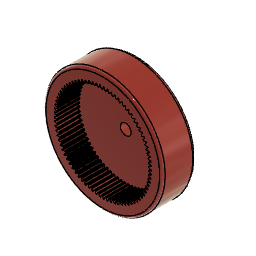
Aquazepp_Zahnkranz2 v37 (Autodesk Fusion 360 design; units mm, degrees)
description: Internal Gear; Module: 1.270000; Number of Teeth: 81; Pressure Angle: 20.000000; Root Fillet Radius: 0.040000; Clearance: 0.000000; Gear Thickness: 2.500000; Outer Diameter: 12.000000;
Autodesk Fusion 360 part; units mm, degrees
(part 1 of 3)
sketch "Skizze1" plane through (0, 0, 0) normal (0, 1, 0) x (1, 0, 0) in component "Internal Gear (81 teeth)"
  spline S0 degree 3 poles (38.2228, -33.6046) (38.0725, -33.5406) (37.9301, -33.4773) (37.7958, -33.4151) knots 0 0 0 0 1 1 1 1
  spline S1 degree 3 poles (40.3792, -34.3646) (39.532, -34.1197) (38.8155, -33.857) (38.2228, -33.6046) knots 0 0 0 0 1 1 1 1
  arc A0 (36.9675, -33.9106) -> (37.3302, -33.511) centre (0, 0) ccw
  arc A1 (36.9675, -33.9106) -> (36.9172, -34.3833) centre (37.2623, -34.181) ccw
  arc A2 (37.7958, -33.4151) -> (37.3302, -33.511) centre (37.6279, -33.7782) ccw
  spline S2 degree 3 poles (37.1472, -34.79) (37.4558, -35.3555) (37.7866, -36.0432) (38.1123, -36.8626) knots 0 0 0 0 1 1 1 1
  spline S3 degree 3 poles (37.5947, -37.3903) (36.7691, -37.0806) (36.0751, -36.7631) (35.5038, -36.4656) knots 0 0 0 0 1 1 1 1
  spline S4 degree 3 poles (36.9172, -34.3833) (36.9921, -34.511) (37.0689, -34.6465) (37.1472, -34.79) knots 0 0 0 0 1 1 1 1
  arc A3 (37.5947, -37.3903) -> (38.1123, -36.8626) centre (0, 0) ccw
  arc A4 (34.2285, -36.6734) -> (34.6211, -36.303) centre (0, 0) ccw
  arc A5 (31.2837, -39.2155) -> (31.161, -39.6748) centre (31.5331, -39.5282) ccw
  arc A6 (31.3657, -42.7504) -> (31.9586, -42.309) centre (0, 0) ccw
  spline S5 degree 3 poles (34.3395, -37.564) (34.6033, -38.1517) (34.8799, -38.863) (35.1411, -39.7052) knots 0 0 0 0 1 1 1 1
  arc A7 (28.1507, -41.5219) -> (27.9928, -41.9702) centre (28.3752, -41.8529) ccw
  spline S6 degree 3 poles (35.5038, -36.4656) (35.3588, -36.3901) (35.2218, -36.3159) (35.0927, -36.2435) knots 0 0 0 0 1 1 1 1
  arc A8 (34.5842, -40.1912) -> (35.1411, -39.7052) centre (0, 0) ccw
  arc A9 (28.1507, -41.5219) -> (28.5958, -41.2166) centre (0, 0) ccw
  spline S7 degree 3 poles (29.4428, -41.5136) (29.3112, -41.4166) (29.1873, -41.3222) (29.071, -41.2307) knots 0 0 0 0 1 1 1 1
  arc A10 (31.2837, -39.2155) -> (31.7038, -38.8767) centre (0, 0) ccw
  arc A11 (32.1786, -38.854) -> (31.7038, -38.8767) centre (31.9566, -39.1867) ccw
  spline S8 degree 3 poles (31.161, -39.6748) (31.2152, -39.8125) (31.2701, -39.9583) (31.3253, -40.1121) knots 0 0 0 0 1 1 1 1
  spline S9 degree 3 poles (34.1418, -37.1407) (34.2065, -37.2738) (34.2726, -37.4149) (34.3395, -37.564) knots 0 0 0 0 1 1 1 1
  arc A12 (35.0927, -36.2435) -> (34.6211, -36.303) centre (34.8972, -36.5925) ccw
  spline S10 degree 3 poles (32.5712, -39.1072) (32.4326, -39.0207) (32.3017, -38.9361) (32.1786, -38.854) knots 0 0 0 0 1 1 1 1
  spline S11 degree 3 poles (31.3657, -42.7504) (30.5979, -42.3168) (29.9613, -41.8959) (29.4428, -41.5136) knots 0 0 0 0 1 1 1 1
  arc A13 (34.2285, -36.6734) -> (34.1418, -37.1407) centre (34.5015, -36.9658) ccw
  spline S12 degree 3 poles (27.9928, -41.9702) (28.0362, -42.1117) (28.0796, -42.2613) (28.1227, -42.419) knots 0 0 0 0 1 1 1 1
  spline S13 degree 3 poles (34.5842, -40.1912) (33.7851, -39.8184) (33.1178, -39.4481) (32.5712, -39.1072) knots 0 0 0 0 1 1 1 1
  spline S14 degree 3 poles (31.3253, -40.1121) (31.5428, -40.7185) (31.7634, -41.449) (31.9586, -42.309) knots 0 0 0 0 1 1 1 1
  arc A14 (29.071, -41.2307) -> (28.5958, -41.2166) centre (28.8238, -41.5452) ccw
  spline S15 degree 3 poles (26.1373, -43.6704) (26.0136, -43.5635) (25.8974, -43.4597) (25.7885, -43.3595) knots 0 0 0 0 1 1 1 1
  arc A15 (24.8484, -43.5785) -> (24.6562, -44.0132) centre (25.0466, -43.9259) ccw
  arc A16 (24.3833, -47.0835) -> (25.0372, -46.739) centre (0, 0) ccw
  arc A17 (25.7885, -43.3595) -> (25.3158, -43.3086) centre (25.5177, -43.6539) ccw
  spline S16 degree 3 poles (24.6562, -44.0132) (24.6885, -44.1577) (24.7203, -44.3102) (24.751, -44.4707) knots 0 0 0 0 1 1 1 1
  arc A18 (21.3967, -45.373) -> (21.1714, -45.7916) centre (21.5673, -45.7348) ccw
  arc A19 (27.9586, -45.0524) -> (28.5839, -44.6583) centre (0, 0) ccw
  spline S17 degree 3 poles (21.1714, -45.7916) (21.1924, -45.9381) (21.2122, -46.0926) (21.2304, -46.255) knots 0 0 0 0 1 1 1 1
  spline S18 degree 3 poles (24.751, -44.4707) (24.8722, -45.1034) (24.9773, -45.8593) (25.0372, -46.739) knots 0 0 0 0 1 1 1 1
  spline S19 degree 3 poles (27.9586, -45.0524) (27.2266, -44.5606) (26.6246, -44.0917) (26.1373, -43.6704) knots 0 0 0 0 1 1 1 1
  spline S20 degree 3 poles (28.1227, -42.419) (28.2926, -43.0404) (28.4559, -43.7858) (28.5839, -44.6583) knots 0 0 0 0 1 1 1 1
  arc A20 (24.8484, -43.5785) -> (25.3158, -43.3086) centre (0, 0) ccw
  spline S21 degree 3 poles (17.5592, -47.2945) (17.5688, -47.4422) (17.5766, -47.5978) (17.5822, -47.7611) knots 0 0 0 0 1 1 1 1
  spline S22 degree 3 poles (20.6613, -48.8314) (20.0142, -48.2325) (19.4918, -47.6761) (19.0754, -47.1846) knots 0 0 0 0 1 1 1 1
  spline S23 degree 3 poles (22.6745, -45.5645) (22.5595, -45.4483) (22.4517, -45.3359) (22.3509, -45.2276) knots 0 0 0 0 1 1 1 1
  spline S24 degree 3 poles (24.3833, -47.0835) (23.6917, -46.5365) (23.1277, -46.0223) (22.6745, -45.5645) knots 0 0 0 0 1 1 1 1
  arc A21 (21.3967, -45.373) -> (21.8836, -45.1402) centre (0, 0) ccw
  arc A22 (20.6613, -48.8314) -> (21.34, -48.5387) centre (0, 0) ccw
  spline S25 degree 3 poles (21.2304, -46.255) (21.3023, -46.8952) (21.3484, -47.6569) (21.34, -48.5387) knots 0 0 0 0 1 1 1 1
  arc A23 (22.3509, -45.2276) -> (21.8836, -45.1402) centre (22.0581, -45.5001) ccw
  arc A24 (17.8163, -46.8946) -> (17.5592, -47.2945) centre (17.9584, -47.2686) ccw
  arc A25 (17.8163, -46.8946) -> (18.3198, -46.7002) centre (0, 0) ccw
  arc A26 (8.8431, -52.28) -> (9.571, -52.1517) centre (0, 0) ccw
  arc A27 (10.3562, -49.0844) -> (10.0404, -49.4397) centre (10.4388, -49.4758) ccw
  arc A28 (6.5214, -49.7393) -> (6.1791, -50.0691) centre (6.5734, -50.1359) ccw
  spline S26 degree 3 poles (17.5822, -47.7611) (17.6042, -48.4049) (17.5912, -49.1679) (17.5145, -50.0464) knots 0 0 0 0 1 1 1 1
  spline S27 degree 3 poles (13.8415, -48.513) (13.8396, -48.661) (13.8353, -48.8167) (13.8282, -48.98) knots 0 0 0 0 1 1 1 1
  arc A29 (14.1288, -48.1342) -> (13.8415, -48.513) centre (14.2414, -48.5181) ccw
  arc A30 (11.3182, -49.1629) -> (10.8837, -48.9701) centre (10.9705, -49.3606) ccw
  spline S28 degree 3 poles (15.3616, -48.5209) (15.266, -48.3884) (15.1768, -48.2606) (15.0939, -48.138) knots 0 0 0 0 1 1 1 1
  spline S29 degree 3 poles (16.8151, -50.2857) (16.2164, -49.6384) (15.7387, -49.0432) (15.3616, -48.5209) knots 0 0 0 0 1 1 1 1
  arc A31 (10.3562, -49.0844) -> (10.8837, -48.9701) centre (0, 0) ccw
  spline S30 degree 3 poles (8.8431, -52.28) (8.3515, -51.5479) (7.9715, -50.8861) (7.6798, -50.3118) knots 0 0 0 0 1 1 1 1
  spline S31 degree 3 poles (12.8678, -51.4375) (12.321, -50.7457) (11.8909, -50.1154) (11.5554, -49.5654) knots 0 0 0 0 1 1 1 1
  spline S32 degree 3 poles (19.0754, -47.1846) (18.9698, -47.0599) (18.871, -46.9394) (18.7789, -46.8236) knots 0 0 0 0 1 1 1 1
  arc A32 (16.8151, -50.2857) -> (17.5145, -50.0464) centre (0, 0) ccw
  arc A33 (15.0939, -48.138) -> (14.6458, -47.9795) centre (14.7626, -48.362) ccw
  spline S33 degree 3 poles (13.8282, -48.98) (13.8002, -49.6236) (13.7282, -50.3833) (13.5836, -51.2532) knots 0 0 0 0 1 1 1 1
  arc A34 (14.1288, -48.1342) -> (14.6458, -47.9795) centre (0, 0) ccw
  spline S34 degree 3 poles (11.5554, -49.5654) (11.4703, -49.4259) (11.3914, -49.2916) (11.3182, -49.1629) knots 0 0 0 0 1 1 1 1
  spline S35 degree 3 poles (10.0404, -49.4397) (10.0271, -49.5871) (10.0108, -49.742) (9.991, -49.9043) knots 0 0 0 0 1 1 1 1
  arc A35 (12.8678, -51.4375) -> (13.5836, -51.2532) centre (0, 0) ccw
  spline S36 degree 3 poles (9.991, -49.9043) (9.9133, -50.5437) (9.7826, -51.2956) (9.571, -52.1517) knots 0 0 0 0 1 1 1 1
  spline S37 degree 3 poles (7.6798, -50.3118) (7.6057, -50.1661) (7.5374, -50.0261) (7.4744, -49.8921) knots 0 0 0 0 1 1 1 1
  arc A36 (7.4744, -49.8921) -> (7.0562, -49.6663) centre (7.1124, -50.0623) ccw
  arc A37 (18.7789, -46.8236) -> (18.3198, -46.7002) centre (18.4659, -47.0726) ccw
  arc A38 (46.1935, -20.2794) -> (45.7794, -20.5129) centre (46.1444, -20.6764) ccw
  spline S38 degree 3 poles (-8.0485, -50.2541) (-8.0745, -50.0928) (-8.0968, -49.9386) (-8.1159, -49.7918) knots 0 0 0 0 1 1 1 1
  spline S39 degree 3 poles (-3.4519, -52.9102) (-3.7614, -52.0844) (-3.9785, -51.3529) (-4.13, -50.7267) knots 0 0 0 0 1 1 1 1
  arc A39 (45.556, -21.0042) -> (45.7794, -20.5129) centre (0, 0) ccw
  arc A40 (44.4831, -23.7981) -> (44.0521, -23.9987) centre (44.4034, -24.1901) ccw
  arc A41 (43.7914, -24.4713) -> (44.0521, -23.9987) centre (0, 0) ccw
  spline S40 degree 3 poles (44.9423, -23.884) (44.7812, -23.8564) (44.6281, -23.8276) (44.4831, -23.7981) knots 0 0 0 0 1 1 1 1
  spline S41 degree 3 poles (4.7652, -52.8081) (4.3318, -52.0401) (4.0043, -51.3508) (3.7579, -50.7556) knots 0 0 0 0 1 1 1 1
  spline S42 degree 3 poles (47.2158, -24.1262) (46.335, -24.0833) (45.5772, -23.9929) (44.9423, -23.884) knots 0 0 0 0 1 1 1 1
  spline S43 degree 3 poles (6.1791, -50.0691) (6.1543, -50.215) (6.1261, -50.3682) (6.0938, -50.5284) knots 0 0 0 0 1 1 1 1
  arc A42 (-5.125, -49.9025) -> (-5.5342, -50.1445) centre (-5.1659, -50.3004) ccw
  spline S44 degree 3 poles (48.8097, -14.4179) (49.3392, -14.7847) (49.9435, -15.2507) (50.6023, -15.8369) knots 0 0 0 0 1 1 1 1
  spline S45 degree 3 poles (44.169, -25.2855) (44.5997, -25.7646) (45.0802, -26.3574) (45.5861, -27.0797) knots 0 0 0 0 1 1 1 1
  spline S46 degree 3 poles (43.8514, -24.9428) (43.9537, -25.0498) (44.0597, -25.164) (44.169, -25.2855) knots 0 0 0 0 1 1 1 1
  arc A43 (2.6474, -50.0951) -> (2.2805, -50.3974) centre (2.6685, -50.4945) ccw
  arc A44 (4.7652, -52.8081) -> (5.5009, -52.7365) centre (0, 0) ccw
  spline S47 degree 3 poles (-0.1866, -50.8942) (-0.2372, -50.7388) (-0.2831, -50.59) (-0.3246, -50.4479) knots 0 0 0 0 1 1 1 1
  arc A45 (-4.233, -50.271) -> (-4.5879, -49.9548) centre (-4.6244, -50.3531) ccw
  spline S48 degree 3 poles (6.0938, -50.5284) (5.9667, -51.16) (5.7781, -51.8994) (5.5009, -52.7365) knots 0 0 0 0 1 1 1 1
  arc A46 (-3.4519, -52.9102) -> (-2.714, -52.9531) centre (0, 0) ccw
  arc A47 (0.6587, -53.0186) -> (1.3977, -53.0042) centre (0, 0) ccw
  arc A48 (-5.125, -49.9025) -> (-4.5879, -49.9548) centre (0, 0) ccw
  spline S49 degree 3 poles (-1.787, -50.8632) (-2.0101, -51.4675) (-2.3107, -52.1689) (-2.714, -52.9531) knots 0 0 0 0 1 1 1 1
  spline S50 degree 3 poles (-5.7231, -50.5718) (-5.9924, -51.157) (-6.3465, -51.833) (-6.8093, -52.5836) knots 0 0 0 0 1 1 1 1
  arc A49 (47.2158, -24.1262) -> (47.5475, -23.4657) centre (0, 0) ccw
  arc A50 (45.2042, -27.7125) -> (45.5861, -27.0797) centre (0, 0) ccw
  spline S51 degree 3 poles (48.0931, -16.6527) (47.9296, -16.6503) (47.7739, -16.6455) (47.6261, -16.6388) knots 0 0 0 0 1 1 1 1
  arc A51 (47.0467, -17.4108) -> (47.1789, -17.8674) centre (47.4218, -17.5496) ccw
  arc A52 (43.7914, -24.4713) -> (43.8514, -24.9428) centre (44.1406, -24.6664) ccw
  arc A53 (42.5051, -27.1736) -> (42.0599, -27.3403) centre (42.3953, -27.5583) ccw
  arc A54 (-0.3246, -50.4479) -> (-0.703, -50.1601) centre (-0.7086, -50.56) ccw
  spline S52 degree 3 poles (-4.13, -50.7267) (-4.1684, -50.5679) (-4.2026, -50.4159) (-4.233, -50.271) knots 0 0 0 0 1 1 1 1
  spline S53 degree 3 poles (-7.5416, -52.4836) (-7.7862, -51.6363) (-7.946, -50.8901) (-8.0485, -50.2541) knots 0 0 0 0 1 1 1 1
  arc A55 (-8.9767, -49.3553) -> (-8.4452, -49.449) centre (0, 0) ccw
  spline S54 degree 3 poles (50.3766, -16.5407) (49.4998, -16.6345) (48.7372, -16.6622) (48.0931, -16.6527) knots 0 0 0 0 1 1 1 1
  spline S55 degree 3 poles (-5.5342, -50.1445) (-5.5919, -50.2807) (-5.6548, -50.4233) (-5.7231, -50.5718) knots 0 0 0 0 1 1 1 1
  arc A56 (45.556, -21.0042) -> (45.6525, -21.4697) centre (45.9193, -21.1717) ccw
  arc A57 (6.5214, -49.7393) -> (7.0562, -49.6663) centre (0, 0) ccw
  arc A58 (-8.1159, -49.7918) -> (-8.4452, -49.449) centre (-8.5125, -49.8433) ccw
  spline S56 degree 3 poles (48.9434, -20.3948) (48.0619, -20.4203) (47.2994, -20.3889) (46.658, -20.3295) knots 0 0 0 0 1 1 1 1
  spline S57 degree 3 poles (45.9956, -21.7867) (46.4621, -22.231) (46.9871, -22.7848) (47.5475, -23.4657) knots 0 0 0 0 1 1 1 1
  spline S58 degree 3 poles (48.4216, -14.1576) (48.5458, -14.2382) (48.6753, -14.3248) (48.8097, -14.4179) knots 0 0 0 0 1 1 1 1
  spline S59 degree 3 poles (2.1599, -50.8487) (1.9843, -51.4685) (1.7389, -52.1911) (1.3977, -53.0042) knots 0 0 0 0 1 1 1 1
  arc A59 (50.3766, -16.5407) -> (50.6023, -15.8369) centre (0, 0) ccw
  spline S60 degree 3 poles (46.658, -20.3295) (46.4952, -20.3145) (46.3404, -20.2976) (46.1935, -20.2794) knots 0 0 0 0 1 1 1 1
  arc A60 (48.9434, -20.3948) -> (49.2229, -19.7105) centre (0, 0) ccw
  spline S61 degree 3 poles (-1.6318, -50.4225) (-1.6788, -50.5629) (-1.7304, -50.7099) (-1.787, -50.8632) knots 0 0 0 0 1 1 1 1
  arc A61 (-1.2426, -50.1496) -> (-0.703, -50.1601) centre (0, 0) ccw
  arc A62 (2.6474, -50.0951) -> (3.1862, -50.0637) centre (0, 0) ccw
  arc A63 (3.5857, -50.3213) -> (3.1862, -50.0637) centre (3.2116, -50.4629) ccw
  arc A64 (-7.5416, -52.4836) -> (-6.8093, -52.5836) centre (0, 0) ccw
  spline S62 degree 3 poles (0.6587, -53.0186) (0.2861, -52.2193) (0.0129, -51.5067) (-0.1866, -50.8942) knots 0 0 0 0 1 1 1 1
  arc A65 (-8.9767, -49.3553) -> (-9.4034, -49.5648) centre (-9.0483, -49.7489) ccw
  arc A66 (47.6261, -16.6388) -> (47.2313, -16.9036) centre (47.6079, -17.0384) ccw
  spline S63 degree 3 poles (2.2805, -50.3974) (2.2445, -50.5409) (2.2045, -50.6915) (2.1599, -50.8487) knots 0 0 0 0 1 1 1 1
  arc A67 (47.0467, -17.4108) -> (47.2313, -16.9036) centre (0, 0) ccw
  spline S64 degree 3 poles (45.6525, -21.4697) (45.7627, -21.5684) (45.8773, -21.674) (45.9956, -21.7867) knots 0 0 0 0 1 1 1 1
  arc A68 (-1.2426, -50.1496) -> (-1.6318, -50.4225) centre (-1.2525, -50.5495) ccw
  spline S65 degree 3 poles (3.7579, -50.7556) (3.6953, -50.6046) (3.6381, -50.4598) (3.5857, -50.3213) knots 0 0 0 0 1 1 1 1
  spline S66 degree 3 poles (47.1789, -17.8674) (47.2965, -17.9573) (47.4189, -18.0537) (47.5456, -18.1569) knots 0 0 0 0 1 1 1 1
  spline S67 degree 3 poles (47.5456, -18.1569) (48.0451, -18.5637) (48.6115, -19.0751) (49.2229, -19.7105) knots 0 0 0 0 1 1 1 1
  spline S68 degree 3 poles (-48.2139, 16.2996) (-48.7288, 16.6867) (-49.3146, 17.1759) (-49.9502, 17.7871) knots 0 0 0 0 1 1 1 1
  arc A69 (-46.3362, 19.2219) -> (-46.5403, 18.7223) centre (0, 0) ccw
  spline S69 degree 3 poles (-38.2227, 32.926) (-38.3024, 33.0507) (-38.3844, 33.1831) (-38.4682, 33.3234) knots 0 0 0 0 1 1 1 1
  arc A70 (-39.0163, 35.9045) -> (-39.513, 35.3571) centre (0, 0) ccw
  spline S70 degree 3 poles (-44.0956, 29.4445) (-43.2258, 29.2997) (-42.4836, 29.1219) (-41.8657, 28.94) knots 0 0 0 0 1 1 1 1
  spline S71 degree 3 poles (-39.0163, 35.9045) (-38.1793, 35.627) (-37.4735, 35.3366) (-36.8911, 35.0615) knots 0 0 0 0 1 1 1 1
  spline S72 degree 3 poles (40.712, -30.5416) (40.5571, -30.4894) (40.4103, -30.4373) (40.2716, -30.3858) knots 0 0 0 0 1 1 1 1
  arc A71 (-46.2447, 25.9389) -> (-46.6018, 25.2917) centre (0, 0) ccw
  arc A72 (-47.6864, 15.5734) -> (-47.8363, 16.0246) centre (-48.0667, 15.6976) ccw
  arc A73 (-43.5268, 25.5051) -> (-43.0884, 25.6888) centre (-43.432, 25.8936) ccw
  spline S73 degree 3 poles (-41.6813, 32.773) (-40.8253, 32.5612) (-40.0992, 32.3265) (-39.4971, 32.0973) knots 0 0 0 0 1 1 1 1
  arc A74 (42.9207, -31.1322) -> (43.3505, -30.5308) centre (0, 0) ccw
  spline S74 degree 3 poles (-47.8363, 16.0246) (-47.9572, 16.1098) (-48.0832, 16.2014) (-48.2139, 16.2996) knots 0 0 0 0 1 1 1 1
  arc A75 (-44.7073, 22.7548) -> (-44.9495, 22.2725) centre (0, 0) ccw
  arc A76 (-38.2546, 32.4517) -> (-38.2227, 32.926) centre (-38.5596, 32.7105) ccw
  arc A77 (-39.0631, 31.9244) -> (-38.6015, 32.0383) centre (-38.9093, 32.2937) ccw
  arc A78 (-44.7073, 22.7548) -> (-44.7856, 23.2237) centre (-45.0638, 22.9363) ccw
  arc A79 (40.2716, -30.3858) -> (39.8148, -30.5174) centre (40.1323, -30.7607) ccw
  spline S75 degree 3 poles (-46.2447, 25.9389) (-45.3663, 25.8619) (-44.6126, 25.7422) (-43.9824, 25.6087) knots 0 0 0 0 1 1 1 1
  spline S76 degree 3 poles (-36.8911, 35.0615) (-36.7433, 34.9917) (-36.6035, 34.9229) (-36.4717, 34.8555) knots 0 0 0 0 1 1 1 1
  spline S77 degree 3 poles (39.7314, -31.8068) (40.0829, -32.3466) (40.466, -33.0066) (40.8543, -33.7984) knots 0 0 0 0 1 1 1 1
  spline S78 degree 3 poles (-46.8058, 19.9868) (-47.2892, 20.4127) (-47.8353, 20.9457) (-48.4216, 21.6044) knots 0 0 0 0 1 1 1 1
  spline S79 degree 3 poles (41.7867, -28.266) (41.8804, -28.3806) (41.9772, -28.5026) (42.0767, -28.6322) knots 0 0 0 0 1 1 1 1
  spline S80 degree 3 poles (-40.6593, 29.865) (-40.7484, 29.9831) (-40.8405, 30.1088) (-40.9349, 30.2422) knots 0 0 0 0 1 1 1 1
  arc A80 (-47.6864, 15.5734) -> (-47.8512, 15.0595) centre (0, 0) ccw
  arc A81 (-40.6543, 29.3897) -> (-40.6593, 29.865) centre (-40.9785, 29.624) ccw
  arc A82 (39.4842, -30.944) -> (39.8148, -30.5174) centre (0, 0) ccw
  arc A83 (-49.6974, 18.4817) -> (-49.9502, 17.7871) centre (0, 0) ccw
  spline S81 degree 3 poles (-49.6974, 18.4817) (-48.8176, 18.5413) (-48.0545, 18.5395) (-47.4112, 18.505) knots 0 0 0 0 1 1 1 1
  arc A84 (-41.4195, 28.8014) -> (-40.9682, 28.9506) centre (-41.2948, 29.1814) ccw
  spline S82 degree 3 poles (42.0767, -28.6322) (42.469, -29.1432) (42.9021, -29.7715) (43.3505, -30.5308) knots 0 0 0 0 1 1 1 1
  spline S83 degree 3 poles (-48.7026, 14.7754) (-48.5392, 14.7793) (-48.3834, 14.7806) (-48.2354, 14.7796) knots 0 0 0 0 1 1 1 1
  spline S84 degree 3 poles (-45.1162, 23.5538) (-45.5652, 24.0158) (-46.0683, 24.5896) (-46.6018, 25.2917) knots 0 0 0 0 1 1 1 1
  spline S85 degree 3 poles (-47.4112, 18.505) (-47.248, 18.4963) (-47.0926, 18.4855) (-46.9451, 18.473) knots 0 0 0 0 1 1 1 1
  arc A85 (-46.3362, 19.2219) -> (-46.4506, 19.6833) centre (-46.7057, 19.3752) ccw
  arc A86 (40.3792, -34.3646) -> (40.8543, -33.7984) centre (0, 0) ccw
  arc A87 (-42.8096, 26.1509) -> (-42.8513, 26.6244) centre (-43.1509, 26.3594) ccw
  arc A88 (-44.0956, 29.4445) -> (-44.5018, 28.8269) centre (0, 0) ccw
  spline S86 degree 3 poles (-43.1553, 26.9792) (-43.5671, 27.4746) (-44.0243, 28.0856) (-44.5018, 28.8269) knots 0 0 0 0 1 1 1 1
  spline S87 degree 3 poles (-42.8513, 26.6244) (-42.9494, 26.7353) (-43.0509, 26.8535) (-43.1553, 26.9792) knots 0 0 0 0 1 1 1 1
  arc A89 (-45.3724, 22.0554) -> (-44.9495, 22.2725) centre (-45.308, 22.4501) ccw
  spline S88 degree 3 poles (-44.7856, 23.2237) (-44.892, 23.3266) (-45.0023, 23.4366) (-45.1162, 23.5538) knots 0 0 0 0 1 1 1 1
  spline S89 degree 3 poles (-41.8657, 28.94) (-41.7089, 28.8939) (-41.5601, 28.8475) (-41.4195, 28.8014) knots 0 0 0 0 1 1 1 1
  spline S90 degree 3 poles (42.9563, -27.2949) (42.7979, -27.2549) (42.6475, -27.2143) (42.5051, -27.1736) knots 0 0 0 0 1 1 1 1
  arc A90 (41.7634, -27.7912) -> (42.0599, -27.3403) centre (0, 0) ccw
  arc A91 (-40.6543, 29.3897) -> (-40.9682, 28.9506) centre (0, 0) ccw
  arc A92 (-42.8096, 26.1509) -> (-43.0884, 25.6888) centre (0, 0) ccw
  spline S91 degree 3 poles (-46.4506, 19.6833) (-46.5646, 19.7777) (-46.6832, 19.8788) (-46.8058, 19.9868) knots 0 0 0 0 1 1 1 1
  arc A93 (41.7634, -27.7912) -> (41.7867, -28.266) centre (42.0964, -28.0128) ccw
  spline S92 degree 3 poles (42.9207, -31.1322) (42.0572, -30.9537) (41.3225, -30.7473) (40.712, -30.5416) knots 0 0 0 0 1 1 1 1
  arc A94 (-48.1157, 22.2773) -> (-48.4216, 21.6044) centre (0, 0) ccw
  arc A95 (-48.2354, 14.7796) -> (-47.8512, 15.0595) centre (-48.2328, 15.1796) ccw
  spline S93 degree 3 poles (-45.8346, 22.1234) (-45.6726, 22.102) (-45.5185, 22.0792) (-45.3724, 22.0554) knots 0 0 0 0 1 1 1 1
  spline S94 degree 3 poles (-48.1157, 22.2773) (-47.234, 22.2686) (-46.4733, 22.2076) (-45.8346, 22.1234) knots 0 0 0 0 1 1 1 1
  spline S95 degree 3 poles (-43.9824, 25.6087) (-43.8225, 25.5749) (-43.6706, 25.5401) (-43.5268, 25.5051) knots 0 0 0 0 1 1 1 1
  spline S96 degree 3 poles (-40.9349, 30.2422) (-41.307, 30.7681) (-41.7155, 31.4127) (-42.1341, 32.1888) knots 0 0 0 0 1 1 1 1
  arc A96 (-46.9451, 18.473) -> (-46.5403, 18.7223) centre (-46.9114, 18.8716) ccw
  arc A97 (-41.6813, 32.773) -> (-42.1341, 32.1888) centre (0, 0) ccw
  spline S97 degree 3 poles (-39.4971, 32.0973) (-39.3444, 32.0391) (-39.1997, 31.9813) (-39.0631, 31.9244) knots 0 0 0 0 1 1 1 1
  arc A98 (-38.2546, 32.4517) -> (-38.6015, 32.0383) centre (0, 0) ccw
  arc A99 (39.4842, -30.944) -> (39.4706, -31.4191) centre (39.799, -31.1907) ccw
  spline S98 degree 3 poles (45.2042, -27.7125) (44.3294, -27.6015) (43.5809, -27.4527) (42.9563, -27.2949) knots 0 0 0 0 1 1 1 1
  spline S99 degree 3 poles (39.4706, -31.4191) (39.5552, -31.5406) (39.6423, -31.6698) (39.7314, -31.8068) knots 0 0 0 0 1 1 1 1
  spline S100 degree 3 poles (-13.4687, 49.0801) (-13.3782, 48.9439) (-13.2941, 48.8128) (-13.216, 48.6871) knots 0 0 0 0 1 1 1 1
  arc A100 (-12.2517, 48.6459) -> (-11.9499, 49.0132) centre (-12.3494, 49.0338) ccw
  spline S101 degree 3 poles (-14.8527, 50.8999) (-14.2794, 50.2298) (-13.8252, 49.6166) (-13.4687, 49.0801) knots 0 0 0 0 1 1 1 1
  arc A101 (-33.661, 37.577) -> (-33.1874, 37.6181) centre (-33.452, 37.9181) ccw
  spline S102 degree 3 poles (-29.7464, 41.2966) (-29.9402, 41.9109) (-30.1323, 42.6495) (-30.294, 43.5164) knots 0 0 0 0 1 1 1 1
  arc A102 (-14.8527, 50.8999) -> (-15.5607, 50.6879) centre (0, 0) ccw
  arc A103 (-13.216, 48.6871) -> (-12.7744, 48.5113) centre (-12.8762, 48.8981) ccw
  arc A104 (-35.6248, 35.3186) -> (-36.0027, 34.9332) centre (0, 0) ccw
  arc A105 (-26.5195, 42.5822) -> (-26.3443, 43.0241) centre (-26.731, 42.9217) ccw
  spline S103 degree 3 poles (-35.7702, 36.2042) (-36.0567, 36.7813) (-36.3606, 37.4812) (-36.6543, 38.3127) knots 0 0 0 0 1 1 1 1
  arc A106 (-29.7396, 40.3991) -> (-30.1725, 40.0768) centre (0, 0) ccw
  arc A107 (-18.7523, 49.5959) -> (-19.4419, 49.3297) centre (0, 0) ccw
  arc A108 (-12.2517, 48.6459) -> (-12.7744, 48.5113) centre (0, 0) ccw
  arc A109 (-10.8636, 51.8978) -> (-11.586, 51.7413) centre (0, 0) ccw
  spline S104 degree 3 poles (-11.9499, 49.0132) (-11.9423, 49.161) (-11.932, 49.3164) (-11.9186, 49.4793) knots 0 0 0 0 1 1 1 1
  arc A110 (-9.4034, 49.5648) -> (-8.9767, 49.3553) centre (-9.0483, 49.7489) ccw
  spline S105 degree 3 poles (-11.9186, 49.4793) (-11.8657, 50.1213) (-11.7642, 50.8777) (-11.586, 51.7413) knots 0 0 0 0 1 1 1 1
  spline S106 degree 3 poles (-29.5991, 40.8532) (-29.648, 40.9929) (-29.6972, 41.1407) (-29.7464, 41.2966) knots 0 0 0 0 1 1 1 1
  arc A111 (-29.7396, 40.3991) -> (-29.5991, 40.8532) centre (-29.9767, 40.7212) ccw
  spline S107 degree 3 poles (-32.9998, 41.502) (-32.2157, 41.0985) (-31.5633, 40.7026) (-31.0303, 40.3407) knots 0 0 0 0 1 1 1 1
  arc A112 (-32.7808, 37.973) -> (-33.1874, 37.6181) centre (0, 0) ccw
  spline S108 degree 3 poles (-26.3443, 43.0241) (-26.3822, 43.1672) (-26.4198, 43.3183) (-26.4568, 43.4775) knots 0 0 0 0 1 1 1 1
  spline S109 degree 3 poles (-27.8109, 42.624) (-27.6832, 42.522) (-27.5631, 42.4229) (-27.4504, 42.327) knots 0 0 0 0 1 1 1 1
  spline S110 degree 3 poles (-38.4682, 33.3234) (-38.7985, 33.8765) (-39.1558, 34.5509) (-39.513, 35.3571) knots 0 0 0 0 1 1 1 1
  arc A113 (-26.5195, 42.5822) -> (-26.9761, 42.2944) centre (0, 0) ccw
  spline S111 degree 3 poles (-26.4568, 43.4775) (-26.6024, 44.105) (-26.7367, 44.8563) (-26.8307, 45.7331) knots 0 0 0 0 1 1 1 1
  arc A114 (-36.4717, 34.8555) -> (-36.0027, 34.9332) centre (-36.2898, 35.2118) ccw
  arc A115 (-24.0878, 44.3269) -> (-23.6175, 44.2577) centre (-23.8058, 44.6106) ccw
  arc A116 (-23.14, 44.5092) -> (-22.931, 44.9362) centre (-23.3245, 44.8641) ccw
  spline S112 degree 3 poles (-22.5393, 47.9936) (-21.8694, 47.4201) (-21.3258, 46.8845) (-20.8907, 46.4094) knots 0 0 0 0 1 1 1 1
  arc A117 (-32.7808, 37.973) -> (-32.6759, 38.4367) centre (-33.0422, 38.2758) ccw
  arc A118 (-36.1166, 38.82) -> (-36.6543, 38.3127) centre (0, 0) ccw
  spline S113 degree 3 poles (-32.6759, 38.4367) (-32.7355, 38.5722) (-32.796, 38.7157) (-32.8571, 38.8673) knots 0 0 0 0 1 1 1 1
  spline S114 degree 3 poles (-32.8571, 38.8673) (-33.098, 39.4648) (-33.3467, 40.1862) (-33.5751, 41.0379) knots 0 0 0 0 1 1 1 1
  spline S115 degree 3 poles (-19.3799, 46.578) (-19.3952, 46.7253) (-19.409, 46.8804) (-19.4209, 47.0434) knots 0 0 0 0 1 1 1 1
  spline S116 degree 3 poles (-18.7523, 49.5959) (-18.1289, 48.9722) (-17.6285, 48.3961) (-17.2315, 47.8887) knots 0 0 0 0 1 1 1 1
  spline S117 degree 3 poles (-31.0303, 40.3407) (-30.8951, 40.2489) (-30.7677, 40.1594) (-30.6478, 40.0725) knots 0 0 0 0 1 1 1 1
  arc A119 (-29.6845, 43.9344) -> (-30.294, 43.5164) centre (0, 0) ccw
  spline S118 degree 3 poles (-34.0631, 37.8148) (-33.9212, 37.7338) (-33.7872, 37.6543) (-33.661, 37.577) knots 0 0 0 0 1 1 1 1
  spline S119 degree 3 poles (-29.6845, 43.9344) (-28.934, 43.4714) (-28.3142, 43.0261) (-27.8109, 42.624) knots 0 0 0 0 1 1 1 1
  arc A120 (-27.4504, 42.327) -> (-26.9761, 42.2944) centre (-27.1912, 42.6317) ccw
  arc A121 (-22.5393, 47.9936) -> (-23.2061, 47.6747) centre (0, 0) ccw
  spline S120 degree 3 poles (-19.4209, 47.0434) (-19.4679, 47.6859) (-19.4845, 48.4489) (-19.4419, 49.3297) knots 0 0 0 0 1 1 1 1
  arc A122 (-26.1906, 46.1026) -> (-26.8307, 45.7331) centre (0, 0) ccw
  arc A123 (-20.5804, 46.0602) -> (-20.1168, 45.9548) centre (-20.2772, 46.3212) ccw
  arc A124 (-23.14, 44.5092) -> (-23.6175, 44.2577) centre (0, 0) ccw
  arc A125 (-30.6478, 40.0725) -> (-30.1725, 40.0768) centre (-30.4131, 40.3963) ccw
  spline S121 degree 3 poles (-36.1166, 38.82) (-35.3037, 38.4784) (-34.6225, 38.1343) (-34.0631, 37.8148) knots 0 0 0 0 1 1 1 1
  arc A126 (-35.6248, 35.3186) -> (-35.5562, 35.7889) centre (-35.9089, 35.6002) ccw
  spline S122 degree 3 poles (-26.1906, 46.1026) (-25.4783, 45.5828) (-24.8949, 45.0909) (-24.4243, 44.651) knots 0 0 0 0 1 1 1 1
  arc A127 (-32.9998, 41.502) -> (-33.5751, 41.0379) centre (0, 0) ccw
  arc A128 (-19.6213, 46.1685) -> (-19.3799, 46.578) centre (-19.7777, 46.5367) ccw
  spline S123 degree 3 poles (-20.8907, 46.4094) (-20.7803, 46.2889) (-20.6769, 46.1724) (-20.5804, 46.0602) knots 0 0 0 0 1 1 1 1
  arc A129 (-19.6213, 46.1685) -> (-20.1168, 45.9548) centre (0, 0) ccw
  spline S124 degree 3 poles (-24.4243, 44.651) (-24.3048, 44.5394) (-24.1928, 44.4312) (-24.0878, 44.3269) knots 0 0 0 0 1 1 1 1
  spline S125 degree 3 poles (-35.5562, 35.7889) (-35.6261, 35.9194) (-35.6976, 36.0578) (-35.7702, 36.2042) knots 0 0 0 0 1 1 1 1
  spline S126 degree 3 poles (-22.931, 44.9362) (-22.9577, 45.0818) (-22.9835, 45.2354) (-23.008, 45.397) knots 0 0 0 0 1 1 1 1
  arc A130 (-15.9846, 47.5502) -> (-15.7122, 47.9398) centre (-16.112, 47.9294) ccw
  spline S127 degree 3 poles (-17.2315, 47.8887) (-17.1308, 47.76) (-17.0368, 47.6358) (-16.9492, 47.5165) knots 0 0 0 0 1 1 1 1
  arc A131 (-16.9492, 47.5165) -> (-16.4952, 47.3755) centre (-16.6267, 47.7532) ccw
  arc A132 (-15.9846, 47.5502) -> (-16.4952, 47.3755) centre (0, 0) ccw
  spline S128 degree 3 poles (-15.717, 48.4069) (-15.714, 49.0511) (-15.6715, 49.8131) (-15.5607, 50.6879) knots 0 0 0 0 1 1 1 1
  spline S129 degree 3 poles (-15.7122, 47.9398) (-15.716, 48.0877) (-15.7178, 48.2435) (-15.717, 48.4069) knots 0 0 0 0 1 1 1 1
  spline S130 degree 3 poles (-23.008, 45.397) (-23.1046, 46.0339) (-23.1803, 46.7933) (-23.2061, 47.6747) knots 0 0 0 0 1 1 1 1
  spline S131 degree 3 poles (-46.6018, -25.2917) (-46.0683, -24.5896) (-45.5652, -24.0158) (-45.1162, -23.5538) knots 0 0 0 0 1 1 1 1
  arc A133 (-49.9398, 7.1488) -> (-49.6035, 7.4847) centre (-49.999, 7.5444) ccw
  spline S132 degree 3 poles (-45.1162, -23.5538) (-45.0023, -23.4366) (-44.892, -23.3266) (-44.7856, -23.2237) knots 0 0 0 0 1 1 1 1
  arc A134 (-48.4216, -21.6044) -> (-48.1157, -22.2773) centre (0, 0) ccw
  spline S133 degree 3 poles (-48.4216, -21.6044) (-47.8353, -20.9457) (-47.2892, -20.4127) (-46.8058, -19.9868) knots 0 0 0 0 1 1 1 1
  spline S134 degree 3 poles (-45.8346, -22.1234) (-46.4733, -22.2076) (-47.234, -22.2686) (-48.1157, -22.2773) knots 0 0 0 0 1 1 1 1
  spline S135 degree 3 poles (-50.6732, 4.7414) (-51.2635, 4.9993) (-51.9463, 5.3402) (-52.7058, 5.7883) knots 0 0 0 0 1 1 1 1
  arc A135 (-46.4506, -19.6833) -> (-46.3362, -19.2219) centre (-46.7057, -19.3752) ccw
  arc A136 (-8.4452, 49.449) -> (-8.9767, 49.3553) centre (0, 0) ccw
  spline S136 degree 3 poles (-49.7011, 10.9569) (-49.5385, 10.9735) (-49.3833, 10.9868) (-49.2357, 10.9973) knots 0 0 0 0 1 1 1 1
  spline S137 degree 3 poles (-51.9563, 10.5805) (-51.0963, 10.7754) (-50.342, 10.8915) (-49.7011, 10.9569) knots 0 0 0 0 1 1 1 1
  arc A137 (-50.3437, 3.2573) -> (-50.0343, 3.6183) centre (-50.4333, 3.6472) ccw
  arc A138 (-48.7499, 11.8313) -> (-48.8743, 11.3061) centre (0, 0) ccw
  arc A139 (-46.5403, -18.7223) -> (-46.3362, -19.2219) centre (0, 0) ccw
  arc A140 (-46.5403, -18.7223) -> (-46.9451, -18.473) centre (-46.9114, -18.8716) ccw
  spline S138 degree 3 poles (-46.8058, -19.9868) (-46.6832, -19.8788) (-46.5646, -19.7777) (-46.4506, -19.6833) knots 0 0 0 0 1 1 1 1
  arc A141 (-4.5879, 49.9548) -> (-4.233, 50.271) centre (-4.6244, 50.3531) ccw
  arc A142 (-43.0884, -25.6888) -> (-43.5268, -25.5051) centre (-43.432, -25.8936) ccw
  spline S139 degree 3 poles (-46.9451, -18.473) (-47.0926, -18.4855) (-47.248, -18.4963) (-47.4112, -18.505) knots 0 0 0 0 1 1 1 1
  spline S140 degree 3 poles (-49.9502, -17.7871) (-49.3146, -17.1759) (-48.7288, -16.6867) (-48.2139, -16.2996) knots 0 0 0 0 1 1 1 1
  arc A143 (-51.9563, 10.5805) -> (-52.0987, 9.8552) centre (0, 0) ccw
  arc A144 (-49.9502, -17.7871) -> (-49.6974, -18.4817) centre (0, 0) ccw
  spline S141 degree 3 poles (-50.2423, 4.5608) (-50.3797, 4.6159) (-50.5235, 4.6759) (-50.6732, 4.7414) knots 0 0 0 0 1 1 1 1
  spline S142 degree 3 poles (-47.4112, -18.505) (-48.0545, -18.5395) (-48.8176, -18.5413) (-49.6974, -18.4817) knots 0 0 0 0 1 1 1 1
  arc A145 (-47.8512, -15.0595) -> (-47.6864, -15.5734) centre (0, 0) ccw
  arc A146 (-4.5879, 49.9548) -> (-5.125, 49.9025) centre (0, 0) ccw
  arc A147 (-8.4452, 49.449) -> (-8.1159, 49.7918) centre (-8.5125, 49.8433) ccw
  spline S143 degree 3 poles (-10.8636, 51.8978) (-10.344, 51.1853) (-9.9387, 50.5388) (-9.6248, 49.9762) knots 0 0 0 0 1 1 1 1
  arc A148 (-49.2357, 10.9973) -> (-48.8743, 11.3061) centre (-49.264, 11.3963) ccw
  spline S144 degree 3 poles (-49.332, 12.5144) (-49.8754, 12.8604) (-50.4973, 13.3027) (-51.1783, 13.8628) knots 0 0 0 0 1 1 1 1
  arc A149 (-49.5201, 8.0179) -> (-49.7378, 8.4405) centre (-49.915, 8.0819) ccw
  spline S145 degree 3 poles (-48.9342, 12.2694) (-49.0614, 12.3451) (-49.1941, 12.4266) (-49.332, 12.5144) knots 0 0 0 0 1 1 1 1
  arc A150 (-43.0884, -25.6888) -> (-42.8096, -26.1509) centre (0, 0) ccw
  spline S146 degree 3 poles (-6.8093, 52.5836) (-6.3465, 51.833) (-5.9924, 51.157) (-5.7231, 50.5718) knots 0 0 0 0 1 1 1 1
  arc A151 (-5.5342, 50.1445) -> (-5.125, 49.9025) centre (-5.1659, 50.3004) ccw
  spline S147 degree 3 poles (-9.6248, 49.9762) (-9.5452, 49.8335) (-9.4715, 49.6962) (-9.4034, 49.5648) knots 0 0 0 0 1 1 1 1
  arc A152 (-44.5018, -28.8269) -> (-44.0956, -29.4445) centre (0, 0) ccw
  spline S148 degree 3 poles (-49.7378, 8.4405) (-49.8705, 8.5061) (-50.0092, 8.5771) (-50.1534, 8.6539) knots 0 0 0 0 1 1 1 1
  spline S149 degree 3 poles (-43.1553, -26.9792) (-43.0509, -26.8535) (-42.9494, -26.7353) (-42.8513, -26.6244) knots 0 0 0 0 1 1 1 1
  spline S150 degree 3 poles (-50.1534, 8.6539) (-50.722, 8.9568) (-51.3763, 9.3495) (-52.0987, 9.8552) knots 0 0 0 0 1 1 1 1
  spline S151 degree 3 poles (-44.5018, -28.8269) (-44.0243, -28.0856) (-43.5671, -27.4746) (-43.1553, -26.9792) knots 0 0 0 0 1 1 1 1
  arc A153 (-52.6199, 6.5225) -> (-52.7058, 5.7883) centre (0, 0) ccw
  arc A154 (-48.7499, 11.8313) -> (-48.9342, 12.2694) centre (-49.1386, 11.9256) ccw
  arc A155 (-42.8513, -26.6244) -> (-42.8096, -26.1509) centre (-43.1509, -26.3594) ccw
  arc A156 (-46.6018, -25.2917) -> (-46.2447, -25.9389) centre (0, 0) ccw
  spline S152 degree 3 poles (-43.9824, -25.6087) (-44.6126, -25.7422) (-45.3663, -25.8619) (-46.2447, -25.9389) knots 0 0 0 0 1 1 1 1
  spline S153 degree 3 poles (-45.3724, -22.0554) (-45.5185, -22.0792) (-45.6726, -22.102) (-45.8346, -22.1234) knots 0 0 0 0 1 1 1 1
  spline S154 degree 3 poles (-8.0485, 50.2541) (-7.946, 50.8901) (-7.7862, 51.6363) (-7.5416, 52.4836) knots 0 0 0 0 1 1 1 1
  spline S155 degree 3 poles (-50.7973, 3.1455) (-50.6392, 3.187) (-50.4879, 3.2242) (-50.3437, 3.2573) knots 0 0 0 0 1 1 1 1
  arc A157 (-49.9925, 4.1564) -> (-50.2423, 4.5608) centre (-50.3911, 4.1895) ccw
  spline S156 degree 3 poles (-50.4008, 7.0725) (-50.2399, 7.1016) (-50.0862, 7.1269) (-49.9398, 7.1488) knots 0 0 0 0 1 1 1 1
  spline S157 degree 3 poles (-5.7231, 50.5718) (-5.6548, 50.4233) (-5.5919, 50.2807) (-5.5342, 50.1445) knots 0 0 0 0 1 1 1 1
  spline S158 degree 3 poles (-50.9801, 14.5749) (-50.1076, 14.7026) (-49.3466, 14.7599) (-48.7026, 14.7754) knots 0 0 0 0 1 1 1 1
  spline S159 degree 3 poles (-43.5268, -25.5051) (-43.6706, -25.5401) (-43.8225, -25.5749) (-43.9824, -25.6087) knots 0 0 0 0 1 1 1 1
  arc A158 (-49.9925, 4.1564) -> (-50.0343, 3.6183) centre (0, 0) ccw
  arc A159 (-44.7856, -23.2237) -> (-44.7073, -22.7548) centre (-45.0638, -22.9363) ccw
  arc A160 (-6.8093, 52.5836) -> (-7.5416, 52.4836) centre (0, 0) ccw
  arc A161 (-44.9495, -22.2725) -> (-44.7073, -22.7548) centre (0, 0) ccw
  arc A162 (-44.9495, -22.2725) -> (-45.3724, -22.0554) centre (-45.308, -22.4501) ccw
  spline S160 degree 3 poles (-52.6199, 6.5225) (-51.7776, 6.7834) (-51.0346, 6.9576) (-50.4008, 7.0725) knots 0 0 0 0 1 1 1 1
  spline S161 degree 3 poles (-8.1159, 49.7918) (-8.0968, 49.9386) (-8.0745, 50.0928) (-8.0485, 50.2541) knots 0 0 0 0 1 1 1 1
  arc A163 (-49.5201, 8.0179) -> (-49.6035, 7.4847) centre (0, 0) ccw
  spline S162 degree 3 poles (-4.233, 50.271) (-4.2026, 50.4159) (-4.1684, 50.5679) (-4.13, 50.7267) knots 0 0 0 0 1 1 1 1
  arc A164 (-50.9801, 14.5749) -> (-51.1783, 13.8628) centre (0, 0) ccw
  arc A165 (-47.8363, -16.0246) -> (-47.6864, -15.5734) centre (-48.0667, -15.6976) ccw
  spline S163 degree 3 poles (-48.7026, -14.7754) (-49.3466, -14.7599) (-50.1076, -14.7026) (-50.9801, -14.5749) knots 0 0 0 0 1 1 1 1
  arc A166 (-51.1783, -13.8628) -> (-50.9801, -14.5749) centre (0, 0) ccw
  arc A167 (-47.8512, -15.0595) -> (-48.2354, -14.7796) centre (-48.2328, -15.1796) ccw
  spline S164 degree 3 poles (-48.2139, -16.2996) (-48.0832, -16.2014) (-47.9572, -16.1098) (-47.8363, -16.0246) knots 0 0 0 0 1 1 1 1
  spline S165 degree 3 poles (-48.2354, -14.7796) (-48.3834, -14.7806) (-48.5392, -14.7793) (-48.7026, -14.7754) knots 0 0 0 0 1 1 1 1
  spline S166 degree 3 poles (-52.9672, 2.4252) (-52.1476, 2.7507) (-51.4203, 2.9819) (-50.7973, 3.1455) knots 0 0 0 0 1 1 1 1
  spline S167 degree 3 poles (-11.9186, -49.4793) (-11.932, -49.3164) (-11.9423, -49.161) (-11.9499, -49.0132) knots 0 0 0 0 1 1 1 1
  spline S168 degree 3 poles (-19.4209, -47.0434) (-19.409, -46.8804) (-19.3952, -46.7253) (-19.3799, -46.578) knots 0 0 0 0 1 1 1 1
  arc A168 (-22.931, -44.9362) -> (-23.14, -44.5092) centre (-23.3245, -44.8641) ccw
  arc A169 (-16.4952, -47.3755) -> (-15.9846, -47.5502) centre (0, 0) ccw
  arc A170 (-50.1643, 0.2699) -> (-50.4447, 0.6537) centre (-50.5643, 0.272) ccw
  spline S169 degree 3 poles (-50.8883, 0.8003) (-51.4968, 1.0117) (-52.2039, 1.2987) (-52.9958, 1.6866) knots 0 0 0 0 1 1 1 1
  arc A171 (-12.7744, -48.5113) -> (-13.216, -48.6871) centre (-12.8762, -48.8981) ccw
  arc A172 (-16.4952, -47.3755) -> (-16.9492, -47.5165) centre (-16.6267, -47.7532) ccw
  spline S170 degree 3 poles (-17.2315, -47.8887) (-17.6285, -48.3961) (-18.1289, -48.9722) (-18.7523, -49.5959) knots 0 0 0 0 1 1 1 1
  arc A173 (-11.586, -51.7413) -> (-10.8636, -51.8978) centre (0, 0) ccw
  arc A174 (-19.4419, -49.3297) -> (-18.7523, -49.5959) centre (0, 0) ccw
  arc A175 (-52.9672, 2.4252) -> (-52.9958, 1.6866) centre (0, 0) ccw
  arc A176 (-12.7744, -48.5113) -> (-12.2517, -48.6459) centre (0, 0) ccw
  arc A177 (-15.5607, -50.6879) -> (-14.8527, -50.8999) centre (0, 0) ccw
  spline S171 degree 3 poles (-13.216, -48.6871) (-13.2941, -48.8128) (-13.3782, -48.9439) (-13.4687, -49.0801) knots 0 0 0 0 1 1 1 1
  spline S172 degree 3 poles (-13.4687, -49.0801) (-13.8252, -49.6166) (-14.2794, -50.2298) (-14.8527, -50.8999) knots 0 0 0 0 1 1 1 1
  arc A178 (-15.7122, -47.9398) -> (-15.9846, -47.5502) centre (-16.112, -47.9294) ccw
  spline S173 degree 3 poles (-19.4419, -49.3297) (-19.4845, -48.4489) (-19.4679, -47.6859) (-19.4209, -47.0434) knots 0 0 0 0 1 1 1 1
  arc A179 (-20.1168, -45.9548) -> (-19.6213, -46.1685) centre (0, 0) ccw
  spline S174 degree 3 poles (-20.8907, -46.4094) (-21.3258, -46.8845) (-21.8694, -47.4201) (-22.5393, -47.9936) knots 0 0 0 0 1 1 1 1
  spline S175 degree 3 poles (-9.4034, -49.5648) (-9.4715, -49.6962) (-9.5452, -49.8335) (-9.6248, -49.9762) knots 0 0 0 0 1 1 1 1
  spline S176 degree 3 poles (-11.586, -51.7413) (-11.7642, -50.8777) (-11.8657, -50.1213) (-11.9186, -49.4793) knots 0 0 0 0 1 1 1 1
  spline S177 degree 3 poles (-16.9492, -47.5165) (-17.0368, -47.6358) (-17.1308, -47.76) (-17.2315, -47.8887) knots 0 0 0 0 1 1 1 1
  spline S178 degree 3 poles (-9.6248, -49.9762) (-9.9387, -50.5388) (-10.344, -51.1853) (-10.8636, -51.8978) knots 0 0 0 0 1 1 1 1
  spline S179 degree 3 poles (-15.717, -48.4069) (-15.7178, -48.2435) (-15.716, -48.0877) (-15.7122, -47.9398) knots 0 0 0 0 1 1 1 1
  spline S180 degree 3 poles (-15.5607, -50.6879) (-15.6715, -49.8131) (-15.714, -49.0511) (-15.717, -48.4069) knots 0 0 0 0 1 1 1 1
  arc A180 (-23.2061, -47.6747) -> (-22.5393, -47.9936) centre (0, 0) ccw
  arc A181 (-20.1168, -45.9548) -> (-20.5804, -46.0602) centre (-20.2772, -46.3212) ccw
  arc A182 (-11.9499, -49.0132) -> (-12.2517, -48.6459) centre (-12.3494, -49.0338) ccw
  arc A183 (-19.3799, -46.578) -> (-19.6213, -46.1685) centre (-19.7777, -46.5367) ccw
  spline S181 degree 3 poles (-20.5804, -46.0602) (-20.6769, -46.1724) (-20.7803, -46.2889) (-20.8907, -46.4094) knots 0 0 0 0 1 1 1 1
  spline S182 degree 3 poles (-23.2061, -47.6747) (-23.1803, -46.7933) (-23.1046, -46.0339) (-23.008, -45.397) knots 0 0 0 0 1 1 1 1
  spline S183 degree 3 poles (-24.4243, -44.651) (-24.8949, -45.0909) (-25.4783, -45.5828) (-26.1906, -46.1026) knots 0 0 0 0 1 1 1 1
  arc A184 (-26.8307, -45.7331) -> (-26.1906, -46.1026) centre (0, 0) ccw
  arc A185 (-26.9761, -42.2944) -> (-27.4504, -42.327) centre (-27.1912, -42.6317) ccw
  arc A186 (-26.9761, -42.2944) -> (-26.5195, -42.5822) centre (0, 0) ccw
  arc A187 (-29.5991, -40.8532) -> (-29.7396, -40.3991) centre (-29.9767, -40.7212) ccw
  spline S184 degree 3 poles (-30.6478, -40.0725) (-30.7677, -40.1594) (-30.8951, -40.2489) (-31.0303, -40.3407) knots 0 0 0 0 1 1 1 1
  spline S185 degree 3 poles (-31.0303, -40.3407) (-31.5633, -40.7026) (-32.2157, -41.0985) (-32.9998, -41.502) knots 0 0 0 0 1 1 1 1
  arc A188 (-30.294, -43.5164) -> (-29.6845, -43.9344) centre (0, 0) ccw
  spline S186 degree 3 poles (-32.8571, -38.8673) (-32.796, -38.7157) (-32.7355, -38.5722) (-32.6759, -38.4367) knots 0 0 0 0 1 1 1 1
  spline S187 degree 3 poles (-36.6543, -38.3127) (-36.3606, -37.4812) (-36.0567, -36.7813) (-35.7702, -36.2042) knots 0 0 0 0 1 1 1 1
  arc A189 (-36.6543, -38.3127) -> (-36.1166, -38.82) centre (0, 0) ccw
  spline S188 degree 3 poles (-34.0631, -37.8148) (-34.6225, -38.1343) (-35.3037, -38.4784) (-36.1166, -38.82) knots 0 0 0 0 1 1 1 1
  spline S189 degree 3 poles (-30.294, -43.5164) (-30.1323, -42.6495) (-29.9402, -41.9109) (-29.7464, -41.2966) knots 0 0 0 0 1 1 1 1
  arc A190 (-33.1874, -37.6181) -> (-33.661, -37.577) centre (-33.452, -37.9181) ccw
  arc A191 (-26.3443, -43.0241) -> (-26.5195, -42.5822) centre (-26.731, -42.9217) ccw
  spline S190 degree 3 poles (-26.8307, -45.7331) (-26.7367, -44.8563) (-26.6024, -44.105) (-26.4568, -43.4775) knots 0 0 0 0 1 1 1 1
  arc A192 (-30.1725, -40.0768) -> (-30.6478, -40.0725) centre (-30.4131, -40.3963) ccw
  arc A193 (-30.1725, -40.0768) -> (-29.7396, -40.3991) centre (0, 0) ccw
  spline S191 degree 3 poles (-24.0878, -44.3269) (-24.1928, -44.4312) (-24.3048, -44.5394) (-24.4243, -44.651) knots 0 0 0 0 1 1 1 1
  spline S192 degree 3 poles (-27.8109, -42.624) (-28.3142, -43.0261) (-28.934, -43.4714) (-29.6845, -43.9344) knots 0 0 0 0 1 1 1 1
  arc A194 (-33.5751, -41.0379) -> (-32.9998, -41.502) centre (0, 0) ccw
  spline S193 degree 3 poles (-23.008, -45.397) (-22.9835, -45.2354) (-22.9577, -45.0818) (-22.931, -44.9362) knots 0 0 0 0 1 1 1 1
  spline S194 degree 3 poles (-33.5751, -41.0379) (-33.3467, -40.1862) (-33.098, -39.4648) (-32.8571, -38.8673) knots 0 0 0 0 1 1 1 1
  spline S195 degree 3 poles (-27.4504, -42.327) (-27.5631, -42.4229) (-27.6832, -42.522) (-27.8109, -42.624) knots 0 0 0 0 1 1 1 1
  arc A195 (-32.6759, -38.4367) -> (-32.7808, -37.973) centre (-33.0422, -38.2758) ccw
  spline S196 degree 3 poles (-29.7464, -41.2966) (-29.6972, -41.1407) (-29.648, -40.9929) (-29.5991, -40.8532) knots 0 0 0 0 1 1 1 1
  arc A196 (-33.1874, -37.6181) -> (-32.7808, -37.973) centre (0, 0) ccw
  spline S197 degree 3 poles (-33.661, -37.577) (-33.7872, -37.6543) (-33.9212, -37.7338) (-34.0631, -37.8148) knots 0 0 0 0 1 1 1 1
  arc A197 (-23.6175, -44.2577) -> (-24.0878, -44.3269) centre (-23.8058, -44.6106) ccw
  spline S198 degree 3 poles (-26.4568, -43.4775) (-26.4198, -43.3183) (-26.3822, -43.1672) (-26.3443, -43.0241) knots 0 0 0 0 1 1 1 1
  arc A198 (-23.6175, -44.2577) -> (-23.14, -44.5092) centre (0, 0) ccw
  spline S199 degree 3 poles (-0.3246, 50.4479) (-0.2831, 50.59) (-0.2372, 50.7388) (-0.1866, 50.8942) knots 0 0 0 0 1 1 1 1
  spline S200 degree 3 poles (1.3977, 53.0042) (1.7389, 52.1911) (1.9843, 51.4685) (2.1599, 50.8487) knots 0 0 0 0 1 1 1 1
  spline S201 degree 3 poles (-40.9349, -30.2422) (-40.8405, -30.1088) (-40.7484, -29.9831) (-40.6593, -29.865) knots 0 0 0 0 1 1 1 1
  arc A199 (-38.6015, -32.0383) -> (-39.0631, -31.9244) centre (-38.9093, -32.2937) ccw
  spline S202 degree 3 poles (-0.1866, 50.8942) (0.0129, 51.5067) (0.2861, 52.2193) (0.6587, 53.0186) knots 0 0 0 0 1 1 1 1
  spline S203 degree 3 poles (-35.7702, -36.2042) (-35.6976, -36.0578) (-35.6261, -35.9194) (-35.5562, -35.7889) knots 0 0 0 0 1 1 1 1
  arc A200 (1.3977, 53.0042) -> (0.6587, 53.0186) centre (0, 0) ccw
  spline S204 degree 3 poles (-1.787, 50.8632) (-1.7304, 50.7099) (-1.6788, 50.5629) (-1.6318, 50.4225) knots 0 0 0 0 1 1 1 1
  spline S205 degree 3 poles (3.5857, 50.3213) (3.6381, 50.4598) (3.6953, 50.6046) (3.7579, 50.7556) knots 0 0 0 0 1 1 1 1
  arc A201 (-38.6015, -32.0383) -> (-38.2546, -32.4517) centre (0, 0) ccw
  spline S206 degree 3 poles (-39.4971, -32.0973) (-40.0992, -32.3265) (-40.8253, -32.5612) (-41.6813, -32.773) knots 0 0 0 0 1 1 1 1
  arc A202 (-40.9682, -28.9506) -> (-40.6543, -29.3897) centre (0, 0) ccw
  spline S207 degree 3 poles (-36.4717, -34.8555) (-36.6035, -34.9229) (-36.7433, -34.9917) (-36.8911, -35.0615) knots 0 0 0 0 1 1 1 1
  arc A203 (-36.0027, -34.9332) -> (-36.4717, -34.8555) centre (-36.2898, -35.2118) ccw
  arc A204 (-38.2227, -32.926) -> (-38.2546, -32.4517) centre (-38.5596, -32.7105) ccw
  arc A205 (-39.513, -35.3571) -> (-39.0163, -35.9045) centre (0, 0) ccw
  spline S208 degree 3 poles (-36.8911, -35.0615) (-37.4735, -35.3366) (-38.1793, -35.627) (-39.0163, -35.9045) knots 0 0 0 0 1 1 1 1
  spline S209 degree 3 poles (-38.4682, -33.3234) (-38.3844, -33.1831) (-38.3024, -33.0507) (-38.2227, -32.926) knots 0 0 0 0 1 1 1 1
  spline S210 degree 3 poles (-39.513, -35.3571) (-39.1558, -34.5509) (-38.7985, -33.8765) (-38.4682, -33.3234) knots 0 0 0 0 1 1 1 1
  arc A206 (-42.1341, -32.1888) -> (-41.6813, -32.773) centre (0, 0) ccw
  arc A207 (-36.0027, -34.9332) -> (-35.6248, -35.3186) centre (0, 0) ccw
  spline S211 degree 3 poles (-42.1341, -32.1888) (-41.7155, -31.4127) (-41.307, -30.7681) (-40.9349, -30.2422) knots 0 0 0 0 1 1 1 1
  arc A208 (-40.9682, -28.9506) -> (-41.4195, -28.8014) centre (-41.2948, -29.1814) ccw
  spline S212 degree 3 poles (-39.0631, -31.9244) (-39.1997, -31.9813) (-39.3444, -32.0391) (-39.4971, -32.0973) knots 0 0 0 0 1 1 1 1
  spline S213 degree 3 poles (-41.4195, -28.8014) (-41.5601, -28.8475) (-41.7089, -28.8939) (-41.8657, -28.94) knots 0 0 0 0 1 1 1 1
  spline S214 degree 3 poles (-41.8657, -28.94) (-42.4836, -29.1219) (-43.2258, -29.2997) (-44.0956, -29.4445) knots 0 0 0 0 1 1 1 1
  arc A209 (-0.703, 50.1601) -> (-1.2426, 50.1496) centre (0, 0) ccw
  arc A210 (-1.6318, 50.4225) -> (-1.2426, 50.1496) centre (-1.2525, 50.5495) ccw
  spline S215 degree 3 poles (-2.714, 52.9531) (-2.3107, 52.1689) (-2.0101, 51.4675) (-1.787, 50.8632) knots 0 0 0 0 1 1 1 1
  arc A211 (-35.5562, -35.7889) -> (-35.6248, -35.3186) centre (-35.9089, -35.6002) ccw
  arc A212 (-40.6593, -29.865) -> (-40.6543, -29.3897) centre (-40.9785, -29.624) ccw
  arc A213 (-0.703, 50.1601) -> (-0.3246, 50.4479) centre (-0.7086, 50.56) ccw
  arc A214 (3.1862, 50.0637) -> (2.6474, 50.0951) centre (0, 0) ccw
  arc A215 (7.0562, 49.6663) -> (7.4744, 49.8921) centre (7.1124, 50.0623) ccw
  spline S216 degree 3 poles (13.8282, 48.98) (13.8353, 48.8167) (13.8396, 48.661) (13.8415, 48.513) knots 0 0 0 0 1 1 1 1
  arc A216 (14.6458, 47.9795) -> (15.0939, 48.138) centre (14.7626, 48.362) ccw
  spline S217 degree 3 poles (11.5554, 49.5654) (11.8909, 50.1154) (12.321, 50.7457) (12.8678, 51.4375) knots 0 0 0 0 1 1 1 1
  spline S218 degree 3 poles (13.5836, 51.2532) (13.7282, 50.3833) (13.8002, 49.6236) (13.8282, 48.98) knots 0 0 0 0 1 1 1 1
  spline S219 degree 3 poles (6.0938, 50.5284) (6.1261, 50.3682) (6.1543, 50.215) (6.1791, 50.0691) knots 0 0 0 0 1 1 1 1
  arc A217 (3.1862, 50.0637) -> (3.5857, 50.3213) centre (3.2116, 50.4629) ccw
  spline S220 degree 3 poles (7.6798, 50.3118) (7.9715, 50.8861) (8.3515, 51.5479) (8.8431, 52.28) knots 0 0 0 0 1 1 1 1
  arc A218 (14.6458, 47.9795) -> (14.1288, 48.1342) centre (0, 0) ccw
  spline S221 degree 3 poles (15.0939, 48.138) (15.1768, 48.2606) (15.266, 48.3884) (15.3616, 48.5209) knots 0 0 0 0 1 1 1 1
  arc A219 (17.5145, 50.0464) -> (16.8151, 50.2857) centre (0, 0) ccw
  arc A220 (9.571, 52.1517) -> (8.8431, 52.28) centre (0, 0) ccw
  spline S222 degree 3 poles (9.571, 52.1517) (9.7826, 51.2956) (9.9133, 50.5437) (9.991, 49.9043) knots 0 0 0 0 1 1 1 1
  spline S223 degree 3 poles (11.3182, 49.1629) (11.3914, 49.2916) (11.4703, 49.4259) (11.5554, 49.5654) knots 0 0 0 0 1 1 1 1
  spline S224 degree 3 poles (17.5145, 50.0464) (17.5912, 49.1679) (17.6042, 48.4049) (17.5822, 47.7611) knots 0 0 0 0 1 1 1 1
  spline S225 degree 3 poles (15.3616, 48.5209) (15.7387, 49.0432) (16.2164, 49.6384) (16.8151, 50.2857) knots 0 0 0 0 1 1 1 1
  spline S226 degree 3 poles (18.7789, 46.8236) (18.871, 46.9394) (18.9698, 47.0599) (19.0754, 47.1846) knots 0 0 0 0 1 1 1 1
  arc A221 (10.0404, 49.4397) -> (10.3562, 49.0844) centre (10.4388, 49.4758) ccw
  arc A222 (10.8837, 48.9701) -> (10.3562, 49.0844) centre (0, 0) ccw
  arc A223 (13.8415, 48.513) -> (14.1288, 48.1342) centre (14.2414, 48.5181) ccw
  spline S227 degree 3 poles (7.4744, 49.8921) (7.5374, 50.0261) (7.6057, 50.1661) (7.6798, 50.3118) knots 0 0 0 0 1 1 1 1
  spline S228 degree 3 poles (5.5009, 52.7365) (5.7781, 51.8994) (5.9667, 51.16) (6.0938, 50.5284) knots 0 0 0 0 1 1 1 1
  spline S229 degree 3 poles (9.991, 49.9043) (10.0108, 49.742) (10.0271, 49.5871) (10.0404, 49.4397) knots 0 0 0 0 1 1 1 1
  arc A224 (5.5009, 52.7365) -> (4.7652, 52.8081) centre (0, 0) ccw
  arc A225 (2.2805, 50.3974) -> (2.6474, 50.0951) centre (2.6685, 50.4945) ccw
  arc A226 (13.5836, 51.2532) -> (12.8678, 51.4375) centre (0, 0) ccw
  arc A227 (10.8837, 48.9701) -> (11.3182, 49.1629) centre (10.9705, 49.3606) ccw
  spline S230 degree 3 poles (2.1599, 50.8487) (2.2045, 50.6915) (2.2445, 50.5409) (2.2805, 50.3974) knots 0 0 0 0 1 1 1 1
  arc A228 (6.1791, 50.0691) -> (6.5214, 49.7393) centre (6.5734, 50.1359) ccw
  arc A229 (7.0562, 49.6663) -> (6.5214, 49.7393) centre (0, 0) ccw
  spline S231 degree 3 poles (3.7579, 50.7556) (4.0043, 51.3508) (4.3318, 52.0401) (4.7652, 52.8081) knots 0 0 0 0 1 1 1 1
  arc A230 (18.3198, 46.7002) -> (18.7789, 46.8236) centre (18.4659, 47.0726) ccw
  arc A231 (21.8836, 45.1402) -> (21.3967, 45.373) centre (0, 0) ccw
  spline S232 degree 3 poles (22.6745, 45.5645) (23.1277, 46.0223) (23.6917, 46.5365) (24.3833, 47.0835) knots 0 0 0 0 1 1 1 1
  spline S233 degree 3 poles (19.0754, 47.1846) (19.4918, 47.6761) (20.0142, 48.2325) (20.6613, 48.8314) knots 0 0 0 0 1 1 1 1
  spline S234 degree 3 poles (24.751, 44.4707) (24.7203, 44.3102) (24.6885, 44.1577) (24.6562, 44.0132) knots 0 0 0 0 1 1 1 1
  arc A232 (25.3158, 43.3086) -> (25.7885, 43.3595) centre (25.5177, 43.6539) ccw
  arc A233 (27.9928, 41.9702) -> (28.1507, 41.5219) centre (28.3752, 41.8529) ccw
  spline S235 degree 3 poles (29.071, 41.2307) (29.1873, 41.3222) (29.3112, 41.4166) (29.4428, 41.5136) knots 0 0 0 0 1 1 1 1
  spline S236 degree 3 poles (29.4428, 41.5136) (29.9613, 41.8959) (30.5979, 42.3168) (31.3657, 42.7504) knots 0 0 0 0 1 1 1 1
  spline S237 degree 3 poles (31.3253, 40.1121) (31.2701, 39.9583) (31.2152, 39.8125) (31.161, 39.6748) knots 0 0 0 0 1 1 1 1
  arc A234 (31.7038, 38.8767) -> (31.2837, 39.2155) centre (0, 0) ccw
  arc A235 (21.8836, 45.1402) -> (22.3509, 45.2276) centre (22.0581, 45.5001) ccw
  spline S238 degree 3 poles (26.1373, 43.6704) (26.6246, 44.0917) (27.2266, 44.5606) (27.9586, 45.0524) knots 0 0 0 0 1 1 1 1
  arc A236 (31.9586, 42.309) -> (31.3657, 42.7504) centre (0, 0) ccw
  arc A237 (24.6562, 44.0132) -> (24.8484, 43.5785) centre (25.0466, 43.9259) ccw
  arc A238 (28.5839, 44.6583) -> (27.9586, 45.0524) centre (0, 0) ccw